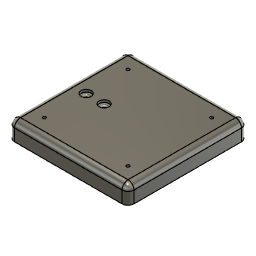
plate A v4 fix v1 (Autodesk Fusion 360 design; units mm, degrees)
Autodesk Fusion 360 part; units mm, degrees
sketch "スケッチ1" plane through (0, 0, 0) normal (0, 1, 0) x (1, 0, 0)
  line L0 (-100, 0) -> (100, 0) construction
  line L1 (0, 100) -> (0, -100) construction
  line L2 (-40, 40) -> (40, 40)
  line L3 (40, 40) -> (40, -40)
  line L4 (40, -40) -> (-40, -40)
  line L5 (-40, -40) -> (-40, 40)
  line L6 (-40, 8) -> (-15, 8)
  line L7 (-15, 8) -> (-15, -8)
  line L8 (-15, -8) -> (-40, -8)
  line L9 (-40, -8) -> (-40, 8)
  circle A0 centre (-35, 0) radius 2.25
  circle A1 centre (-20, 0) radius 2.25
  circle A2 centre (0, 0) radius 35 construction
  circle A3 centre (0, 0) radius 40 construction
  circle A4 centre (-35, 35) radius 1.25
  circle A5 centre (35, 35) radius 1.25
  circle A6 centre (-35, -35) radius 1.25
  circle A7 centre (35, -35) radius 1.25
  circle A8 centre (-35, 0) radius 4.25
  circle A9 centre (-20, 0) radius 4.25
  line L10 (-50, 50) -> (50, 50)
  line L11 (50, 50) -> (50, -50)
  line L12 (50, -50) -> (-50, -50)
  line L13 (-50, -50) -> (-50, 50)
  line L14 (-48, 48) -> (48, 48)
  line L15 (48, 48) -> (48, -48)
  line L16 (48, -48) -> (-48, -48)
  line L17 (-48, -48) -> (-48, 48)
  dimension "d1" = 40
  dimension "d2" = 40
  dimension "d3" = 40
  dimension "d4" = 40
  dimension "d5" = 4.5
  dimension "d6" = 4.5
  dimension "d7" = 15
  dimension "d8" = 5
  dimension "d9" = 25
  dimension "d10" = 8
  dimension "d11" = 8
  dimension "d12" = 70
  dimension "d13" = 80
  dimension "d14" = 2.5
  dimension "d15" = 2.5
  dimension "d16" = 2.5
  dimension "d17" = 2.5
  dimension "d18" = 5
  dimension "d19" = 5
  dimension "d20" = 5
  dimension "d21" = 5
  dimension "d22" = 5
  dimension "d23" = 5
  dimension "d24" = 5
  dimension "d25" = 5
  dimension "d26" = 8.5
  dimension "d27" = 8.5
  dimension "d35" = 50
  dimension "d36" = 50
  dimension "d37" = 50
  dimension "d38" = 50
  dimension "d39" = 2
  dimension "d40" = 2
  dimension "d41" = 2
  dimension "d42" = 2
  constraint horizontal L0
  constraint perpendicular L0 L1
  constraint horizontal L2
  constraint vertical L3
  constraint horizontal L4
  constraint vertical L5
  constraint horizontal L6
  constraint vertical L7
  constraint horizontal L8
  constraint vertical L9
  constraint coincident L5 L6.start
  constraint coincident L0 A0.centre
  constraint coincident L0 A1.centre
  constraint coincident A2.centre A3.centre
  constraint concentric A2 A3
  constraint concentric A0 A8
  constraint concentric A1 A9
  constraint horizontal L10
  constraint vertical L11
  constraint horizontal L12
  constraint vertical L13
  constraint horizontal L14
  constraint vertical L15
  constraint horizontal L16
  constraint vertical L17
  measures "d1" distance of L0 L2
  measures "d2" distance of L0 L4
  measures "d3" distance of L1 L5
  measures "d4" distance of L1 L3
  measures "d5" diameter of A0
  measures "d6" diameter of A1
  measures "d7" distance of A0.centre A1.centre
  measures "d8" distance of L5 A0.centre
  measures "d9" distance of L7 L9
  measures "d10" distance of L0 L6
  measures "d11" distance of L0 L8
  measures "d12" diameter of A2
  measures "d13" diameter of A3
  measures "d14" diameter of A4
  measures "d15" diameter of A5
  measures "d16" diameter of A6
  measures "d17" diameter of A7
  measures "d18" distance of L2 A4.centre
  measures "d19" distance of L5 A4.centre
  measures "d20" distance of L2 A5.centre
  measures "d21" distance of L3 A5.centre
  measures "d22" distance of L4 A6.centre
  measures "d23" distance of L5 A6.centre
  measures "d24" distance of L3 A7.centre
  measures "d25" distance of L4 A7.centre
  measures "d26" diameter of A8
  measures "d27" diameter of A9
  measures "d35" distance of L0 L10
  measures "d36" distance of L0 L12
  measures "d37" distance of L1 L13
  measures "d38" distance of L1 L11
  measures "d39" distance of L12 L16
  measures "d40" distance of L13 L17
  measures "d41" distance of L11 L15
  measures "d42" distance of L10 L14
extrude "押し出し1" add sketch "スケッチ1" against normal blind 3 contours L2 L3 L4 L5 L6 L7 L8 | L14 L15 L16 L17
extrude "押し出し2" add sketch "スケッチ1" against normal blind 8 contours L5 L6 L7 L8 L9
extrude "押し出し3" add sketch "スケッチ1" against normal blind 4 from surface at -4 contours A8 | A9
fillet "フィレット1" radius 2 2 edges at (-38.9624, -4, -1.5369) (-23.9624, -4, -1.5369)
extrude "押し出し4" add sketch "スケッチ1" against normal blind 15 contours L10 L11 L12 L13
sketch "スケッチ2" plane through (0, 0, 0) normal (0, 0, 1) x (1, 0, 0)
fillet "フィレット2" radius 3 8 edges at (48, -9, 48) (48, -9, -48) (-48, -9, -48) (-48, -9, 48) (0, -3, -48) (48, -3, 0) (0, -3, 48) (-48, -3, 0)
fillet "フィレット3" radius 5 8 edges at (0, 0, -50) (50, -7.5, -50) (50, 0, 0) (50, -7.5, 50) (0, 0, 50) (-50, 0, 0) (-50, -7.5, 50) (-50, -7.5, -50)
